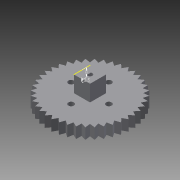
# Autodesk Inventor part: DCMotorStepDownGear
Saved by Autodesk Inventor 2015 (Build 190159000, 159)
## iProperties
Created: 2016-04-11
Part Number: DCMotorStepDownGear
Material: Generic
Document SubType Name: Modeling
Designer: Hatch
Density: 1 g/cm^3
Appearance: Default
Author: Hatch
Autodesk Inventor part; units mm, degrees
ref_plane "YZ Plane" through (0, 0, 0) normal (1, 0, 0) x (0, 1, 0)
ref_plane "XZ Plane" through (0, 0, 0) normal (0, 1, 0) x (-1, 0, 0)
ref_plane "XY Plane" through (0, 0, 0) normal (0, 0, 1) x (1, 0, 0)
sketch "Sketch1" plane through (0, 0, 0) normal (0, 1, 0) x (-1, 0, 0)
  circle A0 centre (0, 0) radius 35
  dimension "d0" = 70
  constraints: 1 centre point, 1 coincident
  measures "d0" diameter of A0
extrude "Gear Base" add sketch "Sketch1" along normal blind 10
sketch "Sketch2" plane through (0, 10, 0) normal (0, 1, 0) x (1, 0, 0)
  arc A0 (-34.5691, 5.4752) -> (-35, 0) centre (0, 0) ccw
  line L0 (0, 0) -> (-34.5691, 5.4752) construction
  line L1 (0, 0) -> (-35, 0) construction
  line L2 (0, 0) -> (-49.4148, 3.889)
  line L3 (0, 0) -> (49.5676, 0) construction
  line L4 (-35, 0) -> (-38.9501, 3.0654)
  line L5 (-38.9501, 3.0654) -> (-34.5691, 5.4752)
  dimension "d3" = 9
  dimension "d4" = 175.5
  dimension "d5" = 5
  constraints: 12 end point, 2 point on circle, 1 centre point, 1 coincident, 1 equal length, 1 horizontal, 1 point on line
  measures "d3" angle of L0 L1
  measures "d4" angle of L3 L2
  measures "d5" distance of L1.end L4.end
extrude "Gear Tooth" add sketch "Sketch2" against normal blind 10
pattern_circular "Circular Pattern1" count 40 over 360 about axis through (0, 0, 0) along (0, 1, 0) of "Gear Tooth"
sketch "Sketch3" plane through (0, 0, 0) normal (0, -1, 0) x (1, 0, 0)
  circle A0 centre (0, 0) radius 10
  dimension "d11" = 20
  constraints: 1 centre point, 1 coincident
  measures "d11" diameter of A0
extrude "Shaft" add sketch "Sketch3" along normal blind 34
sketch "Sketch5" plane through (0, 10, 0) normal (0, 1, 0) x (1, 0, 0)
  line L0 (0, 0) -> (0, 17.5)
  circle A0 centre (0, 17.5) radius 2.6035
  dimension "d15" = 17.5
  dimension "d16" = 5.207
  constraints: 2 end point, 1 centre point, 1 coincident, 1 vertical
  measures "d15" distance of L0.start L0.end
  measures "d16" diameter of A0
extrude "Bolt Hole" cut sketch "Sketch5" against normal through all
pattern_circular "Circular Pattern2" count 4 over 360 about axis through (0, 0, 0) along (0, -1, 0) of "Bolt Hole"
sketch "Sketch7" plane through (0, 10, 0) normal (0, 1, 0) x (1, 0, 0)
  point P0 (0, 0)
sketch "Sketch8" plane through (0, -34, 0) normal (0, -1, 0) x (1, 0, 0)
  circle A0 centre (0, 0) radius 10
  constraints: 1 centre point, 1 coincident
extrude "Extrusion5" cut sketch "Sketch8" against normal blind 34
sketch "Sketch13" plane through (0, 10, 0) normal (0, 1, 0) x (1, 0, 0)
  line L0 (7.5, 7.5) -> (-7.5, 7.5)
  line L1 (-7.5, 7.5) -> (-7.5, -7.5)
  line L2 (-7.5, -7.5) -> (7.5, -7.5)
  line L3 (7.5, -7.5) -> (7.5, 7.5)
  line L4 (7.5, 7.5) -> (-7.5, -7.5) construction
  line L5 (-7.5, 7.5) -> (7.5, -7.5) construction
  point P0 (0, 0)
  dimension "d38" = 15
  dimension "d39" = 15
  constraints: 12 end point, 2 midpoint, 2 parallel, 1 horizontal, 1 perpendicular
  measures "d38" distance of L2.end L1.end
  measures "d39" distance of L1.end L0.end
extrude "Extrusion10" add sketch "Sketch13" along normal blind 15
sketch "Sketch14" plane through (0, 25, 0) normal (0, 1, 0) x (1, 0, 0)
  circle A0 centre (0, 0) radius 2.15
  dimension "d42" = 4.3
  constraints: 1 centre point, 1 coincident
  measures "d42" diameter of A0
extrude "Extrusion11" cut sketch "Sketch14" against normal blind 15
sketch "Sketch15" plane through (-7.5, 10, -7.5) normal (-1, 0, 0) x (0, 0, 1)
  line L0 (15, 15) -> (0, 15) projected
  line L1 (7.5, 15) -> (7.5, 7)
  circle A0 centre (7.5, 7) radius 1.75
  point P0 (7.5, -10)
  dimension "d45" = 8
  dimension "d46" = 3.5
  constraints: 2 end point, 1 centre point, 1 coincident, 1 midpoint, 1 vertical
  measures "d45" distance of L1.start L1.end
  measures "d46" diameter of A0
sketch "Sketch16" plane through (0, 25, 0) normal (0, 1, 0) x (1, 0, 0)
  circle A0 centre (0, 0) radius 2.15
  circle A1 centre (0, 0) radius 2.15 projected
  line L0 (2.15, -0.0117) -> (-1.1, -0.0117)
  line L1 (-1.1, -0.0117) -> (-1.1, 2.15)
  line L2 (-1.1, 2.15) -> (-1.1, 1.8473)
  line L3 (-1.1, 1.8473) -> (-1.1, -2.1527)
  arc A2 (-1.1, 1.8473) -> (-1.1, -1.8473) centre (0, 0) ccw
  dimension "d47" = 3.25
  dimension "d48" = 4
  constraints: 8 end point, 5 point on circle, 3 point on line, 1 centre point, 1 coincident, 1 horizontal, 1 perpendicular, 3 other
  measures "d47" distance of L0.start L0.end
  measures "d48" distance of L2.end L3.end
extrude "Extrusion12" add sketch "Sketch16" against normal blind 15 contours L1 L3 A0
body "Solid1"
